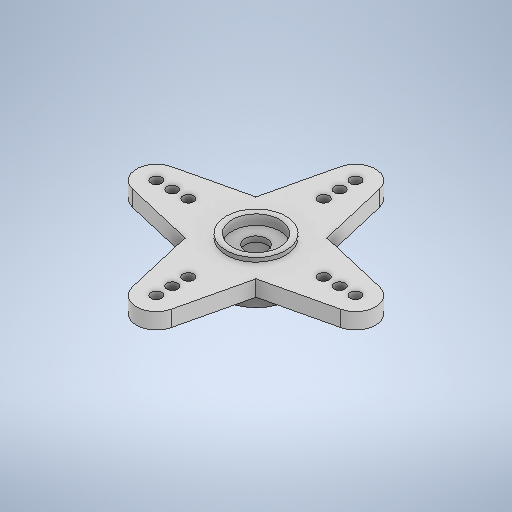
# Autodesk Inventor part: MMAE 232 Assignment 2_Servo Horn 5 - Dylan Tamras
Saved by Autodesk Inventor 2025.2 (Build 292293000, 293)
## iProperties
Created: 2025-01-19
Part Number: MMAE 232 Assignment 2_Servo Horn 5 - Dylan Tamras
Material: Generic
Document SubType Name: Modeling
Designer: Dylan
Density: 1 g/cm^3
Appearance: Default
Author: Dylan
Autodesk Inventor part; units mm, degrees
ref_plane "YZ Plane" through (0, 0, 0) normal (1, 0, 0) x (0, 1, 0)
ref_plane "XZ Plane" through (0, 0, 0) normal (0, 1, 0) x (-1, 0, 0)
ref_plane "XY Plane" through (0, 0, 0) normal (0, 0, 1) x (1, 0, 0)
sketch "Sketch1" plane through (0, 0, 0) normal (0, 1, 0) x (-1, 0, 0)
  circle A0 centre (0, 0) radius 4.45
  circle A1 centre (12.5, 0) radius 2.5
  circle A2 centre (0, -12.5) radius 2.5
  line L0 (4.45, -4.45) -> (13.0693, -2.4343)
  line L1 (4.45, -4.45) -> (2.4343, -13.0693)
  circle A3 centre (12.5, 0) radius 2.5
  circle A4 centre (0, 12.5) radius 2.5
  line L2 (4.45, 4.45) -> (13.0693, 2.4343)
  line L3 (4.45, 4.45) -> (2.4343, 13.0693)
  circle A5 centre (-12.5, 0) radius 2.5
  line L4 (-4.45, -4.45) -> (-13.0693, -2.4343)
  line L5 (-4.45, -4.45) -> (-2.4343, -13.0693)
  line L6 (-4.45, 4.45) -> (-13.0693, 2.4343)
  line L7 (-4.45, 4.45) -> (-2.4343, 13.0693)
  dimension "d2" = 5
  dimension "d0" = 8.9
  constraints: 16 end point, 1 centre point, 1 coincident, 17 other
  measures "d0" diameter of A0
extrude "Extrusion1" add sketch "Sketch1" along normal blind 2 contours A0 | A1 | A1 L0 L1 A2 L5 L4 A5 L6 L7 A4 L3 L2 | A4 | A2 | A5
sketch "Sketch2" plane through (0, 2, 0) normal (0, 1, 0) x (1, 0, 0)
  circle A0 centre (0, 0) radius 3.74
  dimension "d8" = 7.48
  constraints: 1 centre point, 1 coincident
  measures "d8" diameter of A0
extrude "Extrusion2" add sketch "Sketch2" along normal blind 0.5
sketch "Sketch3" plane through (0, 2.5, 0) normal (0, 1, 0) x (1, 0, 0)
  circle A0 centre (0, 0) radius 2.99
  dimension "d11" = 5.98
  constraints: 1 centre point, 1 coincident
  measures "d11" diameter of A0
extrude "Extrusion3" cut sketch "Sketch3" against normal blind 1.25
sketch "Sketch4" plane through (0, 1.25, 0) normal (0, 1, 0) x (1, 0, 0)
  circle A0 centre (0, 0) radius 1.37
  dimension "d14" = 2.74
  constraints: 1 centre point, 1 coincident
  measures "d14" diameter of A0
extrude "Extrusion4" cut sketch "Sketch4" against normal blind 0.69
sketch "Sketch5" plane through (0, 0, 0) normal (0, -1, 0) x (1, 0, 0)
  circle A0 centre (0, 0) radius 4.45
  dimension "d17" = 8.9
  constraints: 1 centre point, 1 coincident
  measures "d17" diameter of A0
extrude "Extrusion5" add sketch "Sketch5" along normal blind 2.44
sketch "Sketch6" plane through (0, -2.44, 0) normal (0, -1, 0) x (1, 0, 0)
  circle A0 centre (0, 0) radius 2.75
  dimension "d20" = 5.5
  constraints: 1 centre point, 1 coincident
  measures "d20" diameter of A0
extrude "Extrusion6" cut sketch "Sketch6" against normal blind 3
sketch "Sketch7" plane through (0, 2, 0) normal (0, 1, 0) x (1, 0, 0)
  circle A0 centre (0, 8.5) radius 0.675
  circle A1 centre (0, 10.5) radius 0.675
  arc A2 (2.4343, 13.0693) -> (-2.4343, 13.0693) centre (0, 12.5) ccw projected
  circle A3 centre (0, 12.5) radius 0.675
  arc A4 (-13.0693, 2.4343) -> (-13.0693, -2.4343) centre (-12.5, 0) ccw projected
  arc A5 (13.0693, -2.4343) -> (13.0693, 2.4343) centre (12.5, 0) ccw projected
  circle A6 centre (0, -8.5) radius 0.675
  circle A7 centre (0, -10.5) radius 0.675
  circle A8 centre (0, -12.5) radius 0.675
  circle A9 centre (0, 0) radius 3.74 projected
  circle A10 centre (8.5, 0) radius 0.675
  circle A11 centre (0, 0) radius 1.37 projected
  circle A12 centre (10.5, 0) radius 0.675
  circle A13 centre (12.5, 0) radius 0.675
  arc A14 (-2.4343, -13.0693) -> (2.4343, -13.0693) centre (0, -12.5) ccw projected
  circle A15 centre (-8.5, 0) radius 0.675
  circle A16 centre (-10.5, 0) radius 0.675
  circle A17 centre (-12.5, 0) radius 0.675
  dimension "d24" = 1.35
  dimension "d26" = 1.35
  dimension "d28" = 1.35
  dimension "d30" = 1.35
  dimension "d32" = 1.35
  dimension "d34" = 1.35
  constraints: 12 centre point, 2 coincident
  measures "d24" diameter of A0
  measures "d26" diameter of A1
  measures "d28" diameter of A3
  measures "d30" diameter of A10
  measures "d32" diameter of A12
  measures "d34" diameter of A13
extrude "Extrusion7" cut sketch "Sketch7" against normal blind 2 contours A0 | A1 | A3 | A6 | A7 | A8 | A10 | A12 | A13 | A15 | A16 | A17
body "Solid1"
